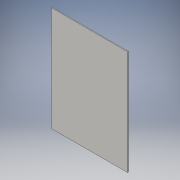
# Autodesk Inventor part: Cabinet Back Sheet
Saved by Autodesk Inventor 2016 (Build 200138000, 138)
## iProperties
Created: 2017-11-05
Part Number: Cabinet Back Sheet
Material: Generic
Document SubType Name: Modeling
Designer: mathaetaes
Density: 1 g/cm^3
Appearance: Default
Author: mathaetaes
Autodesk Inventor part; units mm, degrees
ref_plane "YZ Plane" through (0, 0, 0) normal (1, 0, 0) x (0, 1, 0)
ref_plane "XZ Plane" through (0, 0, 0) normal (0, 1, 0) x (-1, 0, 0)
ref_plane "XY Plane" through (0, 0, 0) normal (0, 0, 1) x (1, 0, 0)
sketch "Sketch1" plane through (0, 0, 0) normal (0, 0, 1) x (1, 0, 0)
  line L0 (153.2956, 0) -> (-427.7294, 0)
  line L1 (-427.7294, 0) -> (-427.7294, 800.1)
  line L2 (-427.7294, 800.1) -> (153.2956, 800.1)
  line L3 (153.2956, 800.1) -> (153.2956, 0)
  point P0 (0, 0)
  dimension "d0" = 800.1
  dimension "d1" = 581.025
  constraints: 8 end point, 2 parallel, 1 horizontal, 1 perpendicular
  measures "d0" distance of L0.end L1.end
  measures "d1" distance of L1.end L2.end
extrude "Board" add sketch "Sketch1" along normal blind 6.35
body "Solid1"
